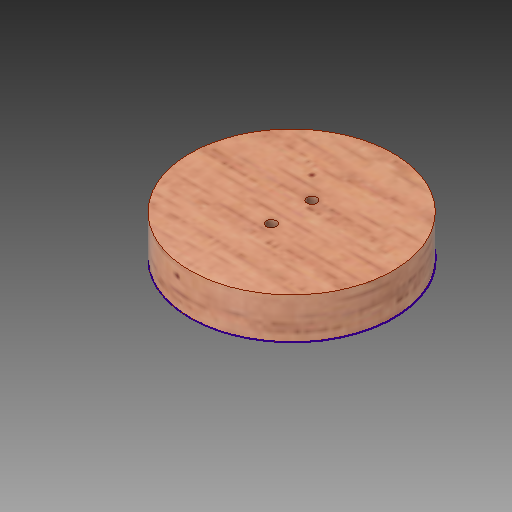
# Autodesk Inventor part: タイヤ
Saved by Autodesk Inventor 2018.2 (Build 222227000, 227)
## iProperties
Created: 2019-04-22
Part Number: タイヤ
Material: 木材 (オーク)
Document SubType Name: Modeling
Designer: Eiji Nishizawa
Density: 0.76 g/cm^3
Appearance: ホワイト オーク材 - ナチュラル 標準の光沢
Author: Eiji Nishizawa
Autodesk Inventor part; units mm, degrees
ref_plane "YZ Plane" through (0, 0, 0) normal (1, 0, 0) x (0, 1, 0)
ref_plane "XZ Plane" through (0, 0, 0) normal (0, 1, 0) x (-1, 0, 0)
ref_plane "XY Plane" through (0, 0, 0) normal (0, 0, 1) x (1, 0, 0)
sketch "スケッチ1" plane through (0, 0, 0) normal (0, 1, 0) x (-1, 0, 0)
  circle A0 centre (0, 0) radius 30
  circle A1 centre (0, 6) radius 1.5
  circle A2 centre (0, -6) radius 1.5
  circle A3 centre (0, 0) radius 3
  dimension "d0" = 60
  dimension "d1" = 9
  dimension "d2" = 6
  dimension "d3" = 3
  dimension "d4" = 3
  dimension "d5" = 6
  dimension "d6" = 6
  constraints: 4 centre point, 2 coincident
  measures "d0" diameter of A0
  measures "d2" distance of A1.centre point (0, 0)
  measures "d3" diameter of A1
  measures "d4" diameter of A2
  measures "d5" distance of point (0, 0) A2.centre
  measures "d6" diameter of A3
extrude "押し出し1" add sketch "スケッチ1" along normal blind 12 contours A0 | A3
extrude "押し出し2" cut sketch "スケッチ1" along normal blind 3 contours A3
